Autodesk Inventor part; units mm, degrees
(part 2 of 16)
  spline S4 degree 3 poles (20.0299, 111.5354) (20.0063, 111.4026) (19.9809, 111.2702) (19.9533, 111.1381) (19.9384, 111.0668) (19.9228, 110.9955) (19.9066, 110.9244) (19.8913, 110.8571) (19.8754, 110.79) (19.8589, 110.723) (19.8433, 110.6597) (19.8272, 110.5966) (19.8105, 110.5336) (19.7948, 110.4744) (19.7786, 110.4154) (19.7618, 110.3565) (19.7461, 110.3013) (19.7299, 110.2462) (19.7133, 110.1914) (19.6977, 110.1402) (19.6817, 110.0892) (19.6653, 110.0383) (19.65, 109.9911) (19.6344, 109.944) (19.6183, 109.8971) (19.6035, 109.8539) (19.5883, 109.8108) (19.5727, 109.7678) (19.5584, 109.7285) (19.5438, 109.6893) (19.5288, 109.6503) (19.5152, 109.6149) (19.5014, 109.5795) (19.4872, 109.5444) (19.4744, 109.5128) (19.4614, 109.4813) (19.4481, 109.45) (19.4305, 109.4086) (19.4123, 109.3675) (19.3937, 109.3265) (19.3896, 109.3173) (19.3854, 109.3081) (19.3813, 109.2989) (19.3774, 109.2899) (19.3735, 109.2809) (19.3697, 109.2718) (19.366, 109.2629) (19.3623, 109.254) (19.3587, 109.2451) (19.3552, 109.2363) (19.3518, 109.2275) (19.3485, 109.2187) (19.3452, 109.21) (19.342, 109.2013) (19.3389, 109.1926) (19.3359, 109.184) (19.3329, 109.1753) (19.3301, 109.1667) (19.3273, 109.1581) (19.3245, 109.1496) (19.3219, 109.1409) (19.3193, 109.1324) (19.3168, 109.1238) (19.3144, 109.1152) (19.3121, 109.1067) (19.3098, 109.0981) (19.3077, 109.0895) (19.3055, 109.0808) (19.3035, 109.0721) (19.3017, 109.0634) (19.2998, 109.0546) (19.298, 109.0458) (19.2964, 109.037) (19.2948, 109.028) (19.2933, 109.019) (19.292, 109.0099) (19.2907, 109.0006) (19.2895, 108.9912) (19.2886, 108.9819) (19.2876, 108.9721) (19.2868, 108.9623) (19.2863, 108.9526) (19.2857, 108.9422) (19.2854, 108.9319) (19.2854, 108.9216) (19.2854, 108.9105) (19.2857, 108.8994) (19.2864, 108.8884) (19.2871, 108.8764) (19.2882, 108.8644) (19.2898, 108.8524) (19.2915, 108.8393) (19.2937, 108.8262) (19.2965, 108.8132) (19.2996, 108.7987) (19.3034, 108.7844) (19.3079, 108.7703) (19.3129, 108.7544) (19.3188, 108.7388) (19.3256, 108.7236) (19.3332, 108.7064) (19.3419, 108.6898) (19.3516, 108.6738) (19.3625, 108.6561) (19.3746, 108.6391) (19.3879, 108.6231) (19.4023, 108.6057) (19.4181, 108.5894) (19.4352, 108.5747) (19.4515, 108.5607) (19.469, 108.5481) (19.4867, 108.5358) (19.5744, 108.4751) (19.6668, 108.4221) (19.7564, 108.3646) (19.8461, 108.3071) (19.9329, 108.2453) (20.0247, 108.191) (20.0432, 108.18) (20.062, 108.1693) (20.0815, 108.1603) (20.102, 108.151) (20.1234, 108.1434) (20.1452, 108.1376) (20.1653, 108.1322) (20.1858, 108.1282) (20.2065, 108.1258) (20.225, 108.1236) (20.2438, 108.1227) (20.2625, 108.1229) (20.2792, 108.1231) (20.2958, 108.1243) (20.3123, 108.1263) (20.327, 108.1281) (20.3416, 108.1307) (20.3561, 108.1339) (20.3691, 108.1368) (20.3819, 108.1402) (20.3946, 108.1442) (20.4061, 108.1477) (20.4174, 108.1517) (20.4286, 108.1561) (20.4389, 108.1601) (20.4491, 108.1644) (20.4592, 108.1691) (20.4686, 108.1734) (20.4779, 108.178) (20.487, 108.1828) (20.4957, 108.1874) (20.5042, 108.1921) (20.5127, 108.1971) (20.5208, 108.2019) (20.5288, 108.2068) (20.5367, 108.2119) (20.5444, 108.2169) (20.552, 108.222) (20.5595, 108.2272) (20.5669, 108.2324) (20.5741, 108.2376) (20.5813, 108.243) (20.5885, 108.2484) (20.5955, 108.2538) (20.6025, 108.2594) (20.6094, 108.2649) (20.6163, 108.2706) (20.6231, 108.2763) (20.6299, 108.282) (20.6366, 108.2879) (20.6433, 108.2938) (20.6501, 108.2998) (20.6567, 108.3058) (20.6633, 108.312) (20.67, 108.3182) (20.6766, 108.3245) (20.6831, 108.3308) (20.6898, 108.3373) (20.6963, 108.3438) (20.7029, 108.3504) (20.7095, 108.3571) (20.7161, 108.3639) (20.7226, 108.3707) (20.7292, 108.3777) (20.7358, 108.3847) (20.7423, 108.3918) (20.7489, 108.3991) (20.7555, 108.4064) (20.7621, 108.4137) (20.7687, 108.4213) (20.7753, 108.4289) (20.7819, 108.4365) (20.8114, 108.4704) (20.8412, 108.5042) (20.8715, 108.5375) (20.8944, 108.5627) (20.9176, 108.5876) (20.9409, 108.6124) (20.967, 108.6399) (20.9933, 108.6673) (21.0198, 108.6944) (21.049, 108.7243) (21.0785, 108.754) (21.1083, 108.7833) (21.1408, 108.8154) (21.1737, 108.8472) (21.2067, 108.8788) (21.2427, 108.913) (21.2789, 108.9468) (21.3154, 108.9804) (21.3548, 109.0166) (21.3945, 109.0524) (21.4345, 109.0879) (21.4774, 109.126) (21.5207, 109.1636) (21.5642, 109.2009) (21.6108, 109.2408) (21.6577, 109.2801) (21.7049, 109.3191) (21.7552, 109.3606) (21.8058, 109.4016) (21.8567, 109.4422) (21.9108, 109.4851) (21.9652, 109.5276) (22.0199, 109.5696) (22.0778, 109.614) (22.136, 109.6579) (22.1946, 109.7012) (22.3031, 109.7814) (22.4128, 109.8598) (22.5237, 109.9366) knots 0 0 0 0 0.057795 0.057795 0.057795 0.089038 0.089038 0.089038 0.118617 0.118617 0.118617 0.14653 0.14653 0.14653 0.172778 0.172778 0.172778 0.19736 0.19736 0.19736 0.220277 0.220277 0.220277 0.241529 0.241529 0.241529 0.261115 0.261115 0.261115 0.279036 0.279036 0.279036 0.295292 0.295292 0.295292 0.309882 0.309882 0.309882 0.329164 0.329164 0.329164 0.333477 0.333477 0.333477 0.337694 0.337694 0.337694 0.34182 0.34182 0.34182 0.345864 0.345864 0.345864 0.349834 0.349834 0.349834 0.353742 0.353742 0.353742 0.3576 0.3576 0.3576 0.361424 0.361424 0.361424 0.365232 0.365232 0.365232 0.369048 0.369048 0.369048 0.372899 0.372899 0.372899 0.376819 0.376819 0.376819 0.380853 0.380853 0.380853 0.385052 0.385052 0.385052 0.389482 0.389482 0.389482 0.394225 0.394225 0.394225 0.399381 0.399381 0.399381 0.405067 0.405067 0.405067 0.411413 0.411413 0.411413 0.418548 0.418548 0.418548 0.426565 0.426565 0.426565 0.435472 0.435472 0.435472 0.445133 0.445133 0.445133 0.45436 0.45436 0.45436 0.5 0.5 0.5 0.54564 0.54564 0.54564 0.554867 0.554867 0.554867 0.564528 0.564528 0.564528 0.573435 0.573435 0.573435 0.581452 0.581452 0.581452 0.588587 0.588587 0.588587 0.594933 0.594933 0.594933 0.600619 0.600619 0.600619 0.605775 0.605775 0.605775 0.610518 0.610518 0.610518 0.614948 0.614948 0.614948 0.619147 0.619147 0.619147 0.623181 0.623181 0.623181 0.627101 0.627101 0.627101 0.630952 0.630952 0.630952 0.634768 0.634768 0.634768 0.638576 0.638576 0.638576 0.6424 0.6424 0.6424 0.646258 0.646258 0.646258 0.650166 0.650166 0.650166 0.654136 0.654136 0.654136 0.65818 0.65818 0.65818 0.662306 0.662306 0.662306 0.666523 0.666523 0.666523 0.670836 0.670836 0.670836 0.690118 0.690118 0.690118 0.704708 0.704708 0.704708 0.720964 0.720964 0.720964 0.738885 0.738885 0.738885 0.758471 0.758471 0.758471 0.779723 0.779723 0.779723 0.80264 0.80264 0.80264 0.827222 0.827222 0.827222 0.85347 0.85347 0.85347 0.881383 0.881383 0.881383 0.910962 0.910962 0.910962 0.942205 0.942205 0.942205 1 1 1 1
  arc A206 (20.0299, 111.5354) -> (19.0221, 112.1094) centre (0.0435, 77.6158) ccw
  spline S5 degree 3 poles (16.3748, 113.4387) (16.3653, 113.3042) (16.3538, 113.1698) (16.3402, 113.0356) (16.3328, 112.9631) (16.3248, 112.8906) (16.3161, 112.8182) (16.3079, 112.7497) (16.2991, 112.6812) (16.2897, 112.6129) (16.2808, 112.5483) (16.2714, 112.4839) (16.2614, 112.4195) (16.2519, 112.359) (16.242, 112.2986) (16.2315, 112.2382) (16.2216, 112.1817) (16.2113, 112.1253) (16.2004, 112.069) (16.1903, 112.0164) (16.1798, 111.964) (16.1687, 111.9117) (16.1585, 111.8632) (16.1478, 111.8147) (16.1367, 111.7664) (16.1265, 111.7219) (16.1159, 111.6774) (16.1049, 111.633) (16.0948, 111.5925) (16.0844, 111.552) (16.0736, 111.5116) (16.0638, 111.4749) (16.0536, 111.4384) (16.0432, 111.4019) (16.0338, 111.3692) (16.0242, 111.3365) (16.0142, 111.3039) (16.001, 111.2609) (15.9872, 111.2181) (15.9731, 111.1754) (15.9699, 111.1658) (15.9667, 111.1563) (15.9636, 111.1467) (15.9606, 111.1373) (15.9577, 111.1279) (15.9549, 111.1185) (15.9521, 111.1093) (15.9494, 111.1001) (15.9468, 111.0908) (15.9442, 111.0817) (15.9417, 111.0726) (15.9393, 111.0635) (15.937, 111.0545) (15.9347, 111.0455) (15.9326, 111.0365) (15.9304, 111.0276) (15.9284, 111.0188) (15.9265, 111.0098) (15.9246, 111.0011) (15.9227, 110.9922) (15.921, 110.9834) (15.9193, 110.9746) (15.9178, 110.9658) (15.9163, 110.957) (15.9148, 110.9483) (15.9135, 110.9395) (15.9123, 110.9307) (15.911, 110.9219) (15.9099, 110.913) (15.909, 110.9042) (15.908, 110.8952) (15.9072, 110.8863) (15.9065, 110.8773) (15.9058, 110.8682) (15.9053, 110.8591) (15.905, 110.8499) (15.9046, 110.8405) (15.9045, 110.8311) (15.9045, 110.8217) (15.9045, 110.8119) (15.9048, 110.8021) (15.9053, 110.7923) (15.9058, 110.782) (15.9066, 110.7717) (15.9077, 110.7614) (15.9088, 110.7504) (15.9103, 110.7394) (15.9121, 110.7285) (15.9141, 110.7166) (15.9164, 110.7048) (15.9192, 110.6931) (15.9223, 110.6802) (15.9259, 110.6674) (15.93, 110.6548) (15.9346, 110.6407) (15.9399, 110.6268) (15.9458, 110.6133) (15.9525, 110.598) (15.96, 110.5831) (15.9683, 110.5687) (15.9777, 110.5524) (15.988, 110.5368) (15.9994, 110.5219) (16.012, 110.5054) (16.0259, 110.4898) (16.0408, 110.4753) (16.0569, 110.4595) (16.0743, 110.445) (16.0928, 110.4321) (16.1105, 110.4199) (16.1293, 110.4092) (16.1482, 110.3988) (16.2417, 110.3476) (16.3392, 110.3045) (16.4343, 110.2567) (16.5295, 110.2089) (16.6223, 110.1565) (16.7192, 110.1121) (16.7388, 110.1031) (16.7586, 110.0944) (16.779, 110.0876) (16.8003, 110.0804) (16.8224, 110.0751) (16.8447, 110.0716) (16.8653, 110.0683) (16.886, 110.0665) (16.9068, 110.0663) (16.9255, 110.066) (16.9443, 110.067) (16.9629, 110.0692) (16.9794, 110.0712) (16.9959, 110.0741) (17.0121, 110.0778) (17.0265, 110.0812) (17.0408, 110.0853) (17.0548, 110.09) (17.0674, 110.0942) (17.0798, 110.099) (17.092, 110.1042) (17.103, 110.1089) (17.1139, 110.1141) (17.1246, 110.1196) (17.1345, 110.1247) (17.1442, 110.1301) (17.1537, 110.1357) (17.1626, 110.141) (17.1713, 110.1465) (17.1799, 110.1523) (17.188, 110.1577) (17.196, 110.1634) (17.2039, 110.1692) (17.2115, 110.1748) (17.219, 110.1805) (17.2263, 110.1864) (17.2334, 110.1922) (17.2404, 110.198) (17.2473, 110.204) (17.2541, 110.2099) (17.2608, 110.2159) (17.2674, 110.222) (17.2739, 110.2281) (17.2804, 110.2343) (17.2867, 110.2405) (17.2931, 110.2467) (17.2993, 110.2531) (17.3054, 110.2595) (17.3116, 110.2659) (17.3177, 110.2724) (17.3237, 110.279) (17.3298, 110.2857) (17.3358, 110.2924) (17.3417, 110.2992) (17.3477, 110.306) (17.3536, 110.313) (17.3595, 110.32) (17.3654, 110.3271) (17.3713, 110.3343) (17.377, 110.3415) (17.3829, 110.3489) (17.3888, 110.3563) (17.3945, 110.3638) (17.4004, 110.3714) (17.4062, 110.3791) (17.4119, 110.3868) (17.4178, 110.3948) (17.4236, 110.4027) (17.4293, 110.4107) (17.4351, 110.4189) (17.4409, 110.4272) (17.4467, 110.4354) (17.4725, 110.4723) (17.4986, 110.5089) (17.5252, 110.5452) (17.5453, 110.5726) (17.5658, 110.5999) (17.5864, 110.6269) (17.6094, 110.6571) (17.6327, 110.687) (17.6563, 110.7168) (17.6822, 110.7496) (17.7085, 110.7821) (17.735, 110.8145) (17.764, 110.8498) (17.7933, 110.8849) (17.8229, 110.9197) (17.8551, 110.9574) (17.8876, 110.9949) (17.9204, 111.0321) (17.9557, 111.0722) (17.9915, 111.112) (18.0276, 111.1515) (18.0663, 111.1938) (18.1054, 111.2358) (18.1448, 111.2774) (18.1869, 111.3219) (18.2295, 111.366) (18.2724, 111.4097) (18.318, 111.4562) (18.364, 111.5022) (18.4105, 111.5479) (18.4597, 111.5963) (18.5094, 111.6442) (18.5594, 111.6918) (18.6123, 111.7419) (18.6657, 111.7916) (18.7195, 111.8409) (18.8189, 111.9319) (18.9198, 112.0214) (19.0221, 112.1094) knots 0 0 0 0 0.057795 0.057795 0.057795 0.089038 0.089038 0.089038 0.118617 0.118617 0.118617 0.14653 0.14653 0.14653 0.172778 0.172778 0.172778 0.19736 0.19736 0.19736 0.220277 0.220277 0.220277 0.241529 0.241529 0.241529 0.261115 0.261115 0.261115 0.279036 0.279036 0.279036 0.295292 0.295292 0.295292 0.309882 0.309882 0.309882 0.329164 0.329164 0.329164 0.333477 0.333477 0.333477 0.337694 0.337694 0.337694 0.34182 0.34182 0.34182 0.345864 0.345864 0.345864 0.349834 0.349834 0.349834 0.353742 0.353742 0.353742 0.3576 0.3576 0.3576 0.361424 0.361424 0.361424 0.365232 0.365232 0.365232 0.369048 0.369048 0.369048 0.372899 0.372899 0.372899 0.376819 0.376819 0.376819 0.380853 0.380853 0.380853 0.385052 0.385052 0.385052 0.389482 0.389482 0.389482 0.394225 0.394225 0.394225 0.399381 0.399381 0.399381 0.405067 0.405067 0.405067 0.411413 0.411413 0.411413 0.418548 0.418548 0.418548 0.426565 0.426565 0.426565 0.435472 0.435472 0.435472 0.445133 0.445133 0.445133 0.45436 0.45436 0.45436 0.5 0.5 0.5 0.54564 0.54564 0.54564 0.554867 0.554867 0.554867 0.564528 0.564528 0.564528 0.573435 0.573435 0.573435 0.581452 0.581452 0.581452 0.588587 0.588587 0.588587 0.594933 0.594933 0.594933 0.600619 0.600619 0.600619 0.605775 0.605775 0.605775 0.610518 0.610518 0.610518 0.614948 0.614948 0.614948 0.619147 0.619147 0.619147 0.623181 0.623181 0.623181 0.627101 0.627101 0.627101 0.630952 0.630952 0.630952 0.634768 0.634768 0.634768 0.638576 0.638576 0.638576 0.6424 0.6424 0.6424 0.646258 0.646258 0.646258 0.650166 0.650166 0.650166 0.654136 0.654136 0.654136 0.65818 0.65818 0.65818 0.662306 0.662306 0.662306 0.666523 0.666523 0.666523 0.670836 0.670836 0.670836 0.690118 0.690118 0.690118 0.704708 0.704708 0.704708 0.720964 0.720964 0.720964 0.738885 0.738885 0.738885 0.758471 0.758471 0.758471 0.779723 0.779723 0.779723 0.80264 0.80264 0.80264 0.827222 0.827222 0.827222 0.85347 0.85347 0.85347 0.881383 0.881383 0.881383 0.910962 0.910962 0.910962 0.942205 0.942205 0.942205 1 1 1 1
  arc A207 (16.3748, 113.4387) -> (15.3125, 113.9042) centre (0.0435, 77.6158) ccw
  spline S6 degree 3 poles (12.5408, 114.9496) (12.5454, 114.8148) (12.548, 114.6799) (12.5485, 114.5451) (12.5488, 114.4722) (12.5484, 114.3993) (12.5473, 114.3264) (12.5463, 114.2573) (12.5447, 114.1883) (12.5425, 114.1193) (12.5404, 114.0542) (12.5378, 113.9892) (12.5345, 113.9241) (12.5315, 113.8629) (12.5279, 113.8018) (12.5237, 113.7407) (12.5199, 113.6834) (12.5155, 113.6262) (12.5106, 113.5691) (12.506, 113.5158) (12.501, 113.4626) (12.4955, 113.4094) (12.4904, 113.36) (12.4849, 113.3108) (12.4789, 113.2615) (12.4733, 113.2162) (12.4674, 113.1708) (12.4611, 113.1256) (12.4553, 113.0841) (12.4492, 113.0428) (12.4427, 113.0015) (12.4368, 112.964) (12.4305, 112.9266) (12.4239, 112.8892) (12.418, 112.8557) (12.4119, 112.8222) (12.4053, 112.7888) (12.3967, 112.7446) (12.3875, 112.7006) (12.3779, 112.6566) (12.3757, 112.6468) (12.3735, 112.637) (12.3715, 112.6271) (12.3695, 112.6175) (12.3675, 112.6078) (12.3657, 112.5982) (12.3639, 112.5887) (12.3622, 112.5792) (12.3606, 112.5698) (12.359, 112.5605) (12.3574, 112.5511) (12.356, 112.5418) (12.3546, 112.5327) (12.3533, 112.5235) (12.3521, 112.5143) (12.3509, 112.5053) (12.3498, 112.4962) (12.3488, 112.4871) (12.3478, 112.4782) (12.347, 112.4692) (12.3462, 112.4603) (12.3454, 112.4514) (12.3448, 112.4425) (12.3442, 112.4336) (12.3437, 112.4247) (12.3433, 112.4158) (12.343, 112.4069) (12.3427, 112.398) (12.3425, 112.3891) (12.3425, 112.3802) (12.3425, 112.3712) (12.3426, 112.3622) (12.3428, 112.3533) (12.3431, 112.3441) (12.3436, 112.335) (12.3442, 112.3259) (12.3448, 112.3165) (12.3456, 112.3071) (12.3467, 112.2977) (12.3477, 112.288) (12.349, 112.2783) (12.3505, 112.2686) (12.3521, 112.2584) (12.354, 112.2482) (12.3561, 112.2381) (12.3584, 112.2272) (12.361, 112.2165) (12.3639, 112.2058) (12.3671, 112.1942) (12.3707, 112.1827) (12.3747, 112.1714) (12.3791, 112.1589) (12.3841, 112.1465) (12.3895, 112.1344) (12.3955, 112.1209) (12.4022, 112.1076) (12.4095, 112.0947) (12.4177, 112.0803) (12.4268, 112.0662) (12.4365, 112.0527) (12.4475, 112.0376) (12.4595, 112.0231) (12.4724, 112.0095) (12.4866, 111.9944) (12.502, 111.9803) (12.5184, 111.9674) (12.5361, 111.9534) (12.5549, 111.9408) (12.5747, 111.93) (12.5936, 111.9196) (12.6133, 111.911) (12.6332, 111.9026) (12.7316, 111.8615) (12.833, 111.8288) (12.9326, 111.7912) (13.0323, 111.7536) (13.13, 111.7112) (13.2311, 111.6772) (13.2515, 111.6703) (13.2721, 111.6637) (13.2931, 111.659) (13.3151, 111.6541) (13.3376, 111.6512) (13.3601, 111.65) (13.3809, 111.6489) (13.4017, 111.6493) (13.4225, 111.6512) (13.4411, 111.6529) (13.4596, 111.6559) (13.4779, 111.66) (13.4941, 111.6637) (13.5102, 111.6683) (13.5259, 111.6737) (13.5399, 111.6786) (13.5537, 111.6841) (13.5671, 111.6902) (13.5792, 111.6958) (13.5911, 111.7018) (13.6026, 111.7083) (13.6131, 111.7141) (13.6234, 111.7204) (13.6335, 111.727) (13.6427, 111.7331) (13.6518, 111.7394) (13.6607, 111.7461) (13.669, 111.7523) (13.6771, 111.7587) (13.685, 111.7653) (13.6926, 111.7715) (13.6999, 111.778) (13.7072, 111.7846) (13.7141, 111.791) (13.7209, 111.7975) (13.7276, 111.8041) (13.7341, 111.8105) (13.7405, 111.8171) (13.7467, 111.8238) (13.7528, 111.8304) (13.7589, 111.837) (13.7648, 111.8438) (13.7706, 111.8505) (13.7764, 111.8573) (13.782, 111.8642) (13.7877, 111.871) (13.7932, 111.878) (13.7987, 111.885) (13.8042, 111.8921) (13.8095, 111.8992) (13.8148, 111.9064) (13.8202, 111.9136) (13.8254, 111.9209) (13.8306, 111.9283) (13.8359, 111.9357) (13.841, 111.9433) (13.8461, 111.9508) (13.8512, 111.9585) (13.8563, 111.9663) (13.8613, 111.9741) (13.8664, 111.982) (13.8714, 111.99) (13.8764, 111.9981) (13.8814, 112.0063) (13.8864, 112.0145) (13.8913, 112.0228) (13.8963, 112.0313) (13.9012, 112.0398) (13.9061, 112.0484) (13.911, 112.0571) (13.9159, 112.0659) (13.9208, 112.0747) (13.9426, 112.1141) (13.9647, 112.1533) (13.9874, 112.1921) (14.0045, 112.2215) (14.022, 112.2508) (14.0397, 112.2798) (14.0595, 112.3122) (14.0795, 112.3445) (14.0998, 112.3765) (14.1222, 112.4118) (14.1449, 112.4469) (14.1679, 112.4819) (14.193, 112.52) (14.2185, 112.558) (14.2443, 112.5957) (14.2723, 112.6366) (14.3007, 112.6773) (14.3295, 112.7177) (14.3605, 112.7613) (14.3919, 112.8046) (14.4236, 112.8476) (14.4577, 112.8938) (14.4922, 112.9396) (14.527, 112.9851) (14.5643, 113.0338) (14.602, 113.082) (14.6401, 113.13) (14.6806, 113.181) (14.7216, 113.2316) (14.763, 113.2819) (14.8069, 113.3352) (14.8513, 113.388) (14.8961, 113.4405) (14.9435, 113.496) (14.9913, 113.551) (15.0396, 113.6055) (15.1291, 113.7065) (15.2201, 113.8061) (15.3125, 113.9042) knots 0 0 0 0 0.057795 0.057795 0.057795 0.089038 0.089038 0.089038 0.118617 0.118617 0.118617 0.14653 0.14653 0.14653 0.172778 0.172778 0.172778 0.19736 0.19736 0.19736 0.220277 0.220277 0.220277 0.241529 0.241529 0.241529 0.261115 0.261115 0.261115 0.279036 0.279036 0.279036 0.295292 0.295292 0.295292 0.309882 0.309882 0.309882 0.329164 0.329164 0.329164 0.333477 0.333477 0.333477 0.337694 0.337694 0.337694 0.34182 0.34182 0.34182 0.345864 0.345864 0.345864 0.349834 0.349834 0.349834 0.353742 0.353742 0.353742 0.3576 0.3576 0.3576 0.361424 0.361424 0.361424 0.365232 0.365232 0.365232 0.369048 0.369048 0.369048 0.372899 0.372899 0.372899 0.376819 0.376819 0.376819 0.380853 0.380853 0.380853 0.385052 0.385052 0.385052 0.389482 0.389482 0.389482 0.394225 0.394225 0.394225 0.399381 0.399381 0.399381 0.405067 0.405067 0.405067 0.411413 0.411413 0.411413 0.418548 0.418548 0.418548 0.426565 0.426565 0.426565 0.435472 0.435472 0.435472 0.445133 0.445133 0.445133 0.45436 0.45436 0.45436 0.5 0.5 0.5 0.54564 0.54564 0.54564 0.554867 0.554867 0.554867 0.564528 0.564528 0.564528 0.573435 0.573435 0.573435 0.581452 0.581452 0.581452 0.588587 0.588587 0.588587 0.594933 0.594933 0.594933 0.600619 0.600619 0.600619 0.605775 0.605775 0.605775 0.610518 0.610518 0.610518 0.614948 0.614948 0.614948 0.619147 0.619147 0.619147 0.623181 0.623181 0.623181 0.627101 0.627101 0.627101 0.630952 0.630952 0.630952 0.634768 0.634768 0.634768 0.638576 0.638576 0.638576 0.6424 0.6424 0.6424 0.646258 0.646258 0.646258 0.650166 0.650166 0.650166 0.654136 0.654136 0.654136 0.65818 0.65818 0.65818 0.662306 0.662306 0.662306 0.666523 0.666523 0.666523 0.670836 0.670836 0.670836 0.690118 0.690118 0.690118 0.704708 0.704708 0.704708 0.720964 0.720964 0.720964 0.738885 0.738885 0.738885 0.758471 0.758471 0.758471 0.779723 0.779723 0.779723 0.80264 0.80264 0.80264 0.827222 0.827222 0.827222 0.85347 0.85347 0.85347 0.881383 0.881383 0.881383 0.910962 0.910962 0.910962 0.942205 0.942205 0.942205 1 1 1 1
  arc A208 (12.5408, 114.9496) -> (11.4357, 115.3015) centre (0.0435, 77.6158) ccw
  spline S7 degree 3 poles (8.5699, 116.0514) (8.5886, 115.9178) (8.6053, 115.784) (8.6198, 115.6499) (8.6277, 115.5774) (8.635, 115.5049) (8.6415, 115.4323) (8.6478, 115.3635) (8.6534, 115.2947) (8.6584, 115.2259) (8.6631, 115.1609) (8.6673, 115.0959) (8.6709, 115.0309) (8.6742, 114.9697) (8.677, 114.9085) (8.6793, 114.8473) (8.6814, 114.79) (8.6831, 114.7326) (8.6842, 114.6753) (8.6852, 114.6218) (8.6858, 114.5684) (8.6858, 114.5149) (8.6859, 114.4653) (8.6856, 114.4157) (8.6847, 114.3661) (8.684, 114.3204) (8.6829, 114.2747) (8.6813, 114.229) (8.6799, 114.1872) (8.6781, 114.1455) (8.6759, 114.1037) (8.674, 114.0658) (8.6717, 114.0279) (8.669, 113.9901) (8.6667, 113.9561) (8.664, 113.9222) (8.661, 113.8883) (8.6571, 113.8435) (8.6525, 113.7987) (8.6475, 113.754) (8.6464, 113.744) (8.6453, 113.734) (8.6443, 113.724) (8.6433, 113.7142) (8.6424, 113.7044) (8.6416, 113.6946) (8.6408, 113.685) (8.64, 113.6754) (8.6394, 113.6658) (8.6388, 113.6563) (8.6383, 113.6469) (8.6378, 113.6375) (8.6374, 113.6282) (8.637, 113.619) (8.6368, 113.6097) (8.6366, 113.6006) (8.6364, 113.5915) (8.6364, 113.5824) (8.6363, 113.5734) (8.6364, 113.5644) (8.6366, 113.5554) (8.6367, 113.5464) (8.637, 113.5375) (8.6374, 113.5286) (8.6378, 113.5197) (8.6383, 113.5108) (8.6389, 113.502) (8.6396, 113.4931) (8.6403, 113.4842) (8.6412, 113.4754) (8.6421, 113.4664) (8.6432, 113.4575) (8.6444, 113.4486) (8.6456, 113.4395) (8.647, 113.4305) (8.6486, 113.4215) (8.6502, 113.4122) (8.652, 113.403) (8.654, 113.3938) (8.6561, 113.3842) (8.6584, 113.3747) (8.6609, 113.3652) (8.6635, 113.3552) (8.6665, 113.3453) (8.6696, 113.3354) (8.6731, 113.3249) (8.6768, 113.3145) (8.6808, 113.3042) (8.6852, 113.293) (8.69, 113.2819) (8.6951, 113.271) (8.7008, 113.259) (8.707, 113.2473) (8.7137, 113.2358) (8.7211, 113.223) (8.7291, 113.2105) (8.7378, 113.1985) (8.7474, 113.1849) (8.7579, 113.1719) (8.769, 113.1595) (8.7815, 113.1456) (8.7949, 113.1325) (8.8091, 113.1203) (8.8249, 113.1067) (8.8417, 113.0944) (8.8593, 113.0832) (8.8784, 113.0712) (8.8984, 113.0605) (8.9192, 113.0519) (8.9391, 113.0436) (8.9596, 113.037) (8.9803, 113.0308) (9.0824, 113.0001) (9.1867, 112.9782) (9.2897, 112.9513) (9.3927, 112.9243) (9.4944, 112.8923) (9.5985, 112.869) (9.6195, 112.8643) (9.6406, 112.86) (9.662, 112.8575) (9.6844, 112.8549) (9.7071, 112.8543) (9.7296, 112.8555) (9.7504, 112.8566) (9.7711, 112.8592) (9.7915, 112.8632) (9.8098, 112.8669) (9.828, 112.8718) (9.8457, 112.8778) (9.8615, 112.8831) (9.8769, 112.8894) (9.892, 112.8964) (9.9054, 112.9027) (9.9186, 112.9097) (9.9313, 112.9172) (9.9427, 112.9239) (9.9539, 112.9312) (9.9647, 112.9388) (9.9745, 112.9458) (9.9841, 112.9531) (9.9934, 112.9607) (10.002, 112.9677) (10.0104, 112.975) (10.0185, 112.9825) (10.0261, 112.9895) (10.0335, 112.9967) (10.0407, 113.0041) (10.0475, 113.0112) (10.0542, 113.0183) (10.0607, 113.0257) (10.0669, 113.0327) (10.073, 113.0399) (10.079, 113.0472) (10.0848, 113.0543) (10.0904, 113.0615) (10.0959, 113.0688) (10.1013, 113.076) (10.1066, 113.0832) (10.1118, 113.0906) (10.1169, 113.0978) (10.1219, 113.1052) (10.1269, 113.1126) (10.1317, 113.1201) (10.1365, 113.1275) (10.1412, 113.1351) (10.1459, 113.1427) (10.1505, 113.1503) (10.1551, 113.158) (10.1596, 113.1658) (10.1641, 113.1736) (10.1685, 113.1815) (10.1729, 113.1894) (10.1772, 113.1975) (10.1815, 113.2055) (10.1858, 113.2137) (10.19, 113.222) (10.1942, 113.2302) (10.1984, 113.2387) (10.2026, 113.2471) (10.2067, 113.2557) (10.2108, 113.2643) (10.2149, 113.2731) (10.2189, 113.2818) (10.223, 113.2908) (10.227, 113.2998) (10.2309, 113.3088) (10.2349, 113.318) (10.2389, 113.3273) (10.2428, 113.3365) (10.2604, 113.378) (10.2783, 113.4192) (10.2968, 113.4603) (10.3108, 113.4913) (10.3251, 113.5222) (10.3397, 113.5529) (10.3559, 113.5872) (10.3725, 113.6214) (10.3893, 113.6554) (10.4079, 113.6928) (10.4268, 113.7301) (10.446, 113.7673) (10.467, 113.8079) (10.4884, 113.8482) (10.5101, 113.8885) (10.5337, 113.9321) (10.5577, 113.9755) (10.5821, 114.0187) (10.6083, 114.0653) (10.635, 114.1116) (10.6621, 114.1577) (10.6912, 114.2072) (10.7207, 114.2564) (10.7506, 114.3053) (10.7826, 114.3576) (10.815, 114.4095) (10.8479, 114.4612) (10.8828, 114.5162) (10.9183, 114.5708) (10.9542, 114.6251) (10.9923, 114.6827) (11.0309, 114.7399) (11.07, 114.7968) (11.1113, 114.8569) (11.1532, 114.9166) (11.1955, 114.9759) (11.2739, 115.0857) (11.354, 115.1942) (11.4357, 115.3015) knots 0 0 0 0 0.057795 0.057795 0.057795 0.089038 0.089038 0.089038 0.118617 0.118617 0.118617 0.14653 0.14653 0.14653 0.172778 0.172778 0.172778 0.19736 0.19736 0.19736 0.220277 0.220277 0.220277 0.241529 0.241529 0.241529 0.261115 0.261115 0.261115 0.279036 0.279036 0.279036 0.295292 0.295292 0.295292 0.309882 0.309882 0.309882 0.329164 0.329164 0.329164 0.333477 0.333477 0.333477 0.337694 0.337694 0.337694 0.34182 0.34182 0.34182 0.345864 0.345864 0.345864 0.349834 0.349834 0.349834 0.353742 0.353742 0.353742 0.3576 0.3576 0.3576 0.361424 0.361424 0.361424 0.365232 0.365232 0.365232 0.369048 0.369048 0.369048 0.372899 0.372899 0.372899 0.376819 0.376819 0.376819 0.380853 0.380853 0.380853 0.385052 0.385052 0.385052 0.389482 0.389482 0.389482 0.394225 0.394225 0.394225 0.399381 0.399381 0.399381 0.405067 0.405067 0.405067 0.411413 0.411413 0.411413 0.418548 0.418548 0.418548 0.426565 0.426565 0.426565 0.435472 0.435472 0.435472 0.445133 0.445133 0.445133 0.45436 0.45436 0.45436 0.5 0.5 0.5 0.54564 0.54564 0.54564 0.554867 0.554867 0.554867 0.564528 0.564528 0.564528 0.573435 0.573435 0.573435 0.581452 0.581452 0.581452 0.588587 0.588587 0.588587 0.594933 0.594933 0.594933 0.600619 0.600619 0.600619 0.605775 0.605775 0.605775 0.610518 0.610518 0.610518 0.614948 0.614948 0.614948 0.619147 0.619147 0.619147 0.623181 0.623181 0.623181 0.627101 0.627101 0.627101 0.630952 0.630952 0.630952 0.634768 0.634768 0.634768 0.638576 0.638576 0.638576 0.6424 0.6424 0.6424 0.646258 0.646258 0.646258 0.650166 0.650166 0.650166 0.654136 0.654136 0.654136 0.65818 0.65818 0.65818 0.662306 0.662306 0.662306 0.666523 0.666523 0.666523 0.670836 0.670836 0.670836 0.690118 0.690118 0.690118 0.704708 0.704708 0.704708 0.720964 0.720964 0.720964 0.738885 0.738885 0.738885 0.758471 0.758471 0.758471 0.779723 0.779723 0.779723 0.80264 0.80264 0.80264 0.827222 0.827222 0.827222 0.85347 0.85347 0.85347 0.881383 0.881383 0.881383 0.910962 0.910962 0.910962 0.942205 0.942205 0.942205 1 1 1 1
  arc A209 (8.5699, 116.0514) -> (7.4341, 116.2859) centre (0.0435, 77.6158) ccw
  spline S8 degree 3 poles (4.5056, 116.7321) (4.5381, 116.6012) (4.5687, 116.4698) (4.5972, 116.338) (4.6126, 116.2668) (4.6274, 116.1954) (4.6415, 116.1238) (4.6549, 116.0561) (4.6677, 115.9883) (4.6799, 115.9203) (4.6914, 115.8562) (4.7023, 115.792) (4.7126, 115.7277) (4.7224, 115.6672) (4.7316, 115.6067) (4.7402, 115.546) (4.7483, 115.4893) (4.756, 115.4324) (4.763, 115.3755) (4.7697, 115.3224) (4.7758, 115.2693) (4.7815, 115.2161) (4.7867, 115.1668) (4.7916, 115.1174) (4.796, 115.068) (4.8, 115.0225) (4.8036, 114.9769) (4.8069, 114.9314) (4.8098, 114.8896) (4.8124, 114.8479) (4.8146, 114.8061) (4.8166, 114.7683) (4.8183, 114.7304) (4.8196, 114.6925) (4.8208, 114.6584) (4.8218, 114.6244) (4.8223, 114.5904) (4.8231, 114.5454) (4.8232, 114.5004) (4.8229, 114.4554) (4.8229, 114.4453) (4.8228, 114.4352) (4.8228, 114.4252) (4.8228, 114.4153) (4.823, 114.4055) (4.8232, 114.3957) (4.8234, 114.386) (4.8237, 114.3764) (4.8241, 114.3668) (4.8244, 114.3574) (4.8249, 114.3479) (4.8254, 114.3385) (4.826, 114.3293) (4.8266, 114.32) (4.8273, 114.3108) (4.828, 114.3017) (4.8288, 114.2926) (4.8298, 114.2835) (4.8307, 114.2746) (4.8317, 114.2656) (4.8328, 114.2567) (4.8339, 114.2478) (4.8351, 114.239) (4.8364, 114.2302) (4.8377, 114.2214) (4.8391, 114.2126) (4.8407, 114.2039) (4.8423, 114.1951) (4.844, 114.1864) (4.8458, 114.1776) (4.8476, 114.1688) (4.8496, 114.1601) (4.8517, 114.1513) (4.8539, 114.1425) (4.8562, 114.1336) (4.8587, 114.1248) (4.8613, 114.1158) (4.8641, 114.1068) (4.867, 114.0978) (4.8701, 114.0885) (4.8734, 114.0793) (4.8769, 114.0701) (4.8805, 114.0605) (4.8845, 114.0509) (4.8887, 114.0414) (4.8932, 114.0313) (4.8979, 114.0213) (4.903, 114.0115) (4.9086, 114.0008) (4.9145, 113.9903) (4.9208, 113.9801) (4.9277, 113.9687) (4.935, 113.9577) (4.9429, 113.947) (4.9516, 113.935) (4.9609, 113.9234) (4.9707, 113.9123) (4.9818, 113.8999) (4.9935, 113.888) (5.0059, 113.8769) (5.0198, 113.8643) (5.0345, 113.8527) (5.0499, 113.842) (5.067, 113.8302) (5.085, 113.8197) (5.1036, 113.8104) (5.1239, 113.8004) (5.1449, 113.792) (5.1665, 113.7855) (5.1871, 113.7793) (5.2083, 113.7749) (5.2294, 113.7709) (5.3342, 113.7511) (5.4402, 113.7402) (5.5455, 113.7242) (5.6508, 113.7082) (5.7552, 113.687) (5.8612, 113.6747) (5.8826, 113.6722) (5.904, 113.6701) (5.9256, 113.6698) (5.9481, 113.6696) (5.9707, 113.6714) (5.993, 113.6749) (6.0136, 113.6782) (6.0339, 113.6829) (6.0537, 113.6891) (6.0716, 113.6947) (6.0891, 113.7014) (6.1061, 113.7092) (6.1212, 113.7162) (6.136, 113.724) (6.1502, 113.7326) (6.1629, 113.7403) (6.1752, 113.7485) (6.1871, 113.7574) (6.1978, 113.7653) (6.2081, 113.7736) (6.2181, 113.7824) (6.2272, 113.7903) (6.2359, 113.7986) (6.2444, 113.8071) (6.2522, 113.815) (6.2597, 113.8231) (6.267, 113.8314) (6.2738, 113.8392) (6.2804, 113.8471) (6.2868, 113.8553) (6.2929, 113.863) (6.2988, 113.8708) (6.3045, 113.8788) (6.31, 113.8864) (6.3153, 113.8942) (6.3204, 113.9021) (6.3254, 113.9097) (6.3303, 113.9175) (6.335, 113.9253) (6.3396, 113.933) (6.3441, 113.9408) (6.3485, 113.9487) (6.3529, 113.9564) (6.3571, 113.9643) (6.3612, 113.9722) (6.3653, 113.9801) (6.3693, 113.988) (6.3731, 113.996) (6.377, 114.004) (6.3808, 114.0121) (6.3845, 114.0203) (6.3882, 114.0284) (6.3918, 114.0367) (6.3954, 114.045) (6.3989, 114.0534) (6.4024, 114.0618) (6.4058, 114.0703) (6.4092, 114.0789) (6.4126, 114.0875) (6.4159, 114.0962) (6.4192, 114.105) (6.4224, 114.1139) (6.4256, 114.1228) (6.4288, 114.1318) (6.432, 114.1409) (6.435, 114.1501) (6.4382, 114.1594) (6.4412, 114.1687) (6.4442, 114.1781) (6.4472, 114.1877) (6.4501, 114.1974) (6.4531, 114.207) (6.4662, 114.25) (6.4797, 114.2929) (6.4938, 114.3357) (6.5045, 114.368) (6.5155, 114.4002) (6.5268, 114.4323) (6.5394, 114.4681) (6.5523, 114.5038) (6.5655, 114.5394) (6.58, 114.5786) (6.5949, 114.6176) (6.6102, 114.6566) (6.6268, 114.6991) (6.6439, 114.7416) (6.6613, 114.7838) (6.6802, 114.8297) (6.6995, 114.8753) (6.7192, 114.9208) (6.7404, 114.9699) (6.7621, 115.0188) (6.7843, 115.0675) (6.808, 115.1197) (6.8322, 115.1717) (6.8568, 115.2235) (6.8832, 115.2788) (6.91, 115.3339) (6.9373, 115.3887) (6.9663, 115.447) (6.9959, 115.5051) (7.0259, 115.5629) (7.0578, 115.6241) (7.0902, 115.685) (7.1231, 115.7457) (7.1579, 115.8098) (7.1933, 115.8735) (7.2292, 115.937) (7.2957, 116.0543) (7.364, 116.1706) (7.4341, 116.2859) knots 0 0 0 0 0.057795 0.057795 0.057795 0.089038 0.089038 0.089038 0.118617 0.118617 0.118617 0.14653 0.14653 0.14653 0.172778 0.172778 0.172778 0.19736 0.19736 0.19736 0.220277 0.220277 0.220277 0.241529 0.241529 0.241529 0.261115 0.261115 0.261115 0.279036 0.279036 0.279036 0.295292 0.295292 0.295292 0.309882 0.309882 0.309882 0.329164 0.329164 0.329164 0.333477 0.333477 0.333477 0.337694 0.337694 0.337694 0.34182 0.34182 0.34182 0.345864 0.345864 0.345864 0.349834 0.349834 0.349834 0.353742 0.353742 0.353742 0.3576 0.3576 0.3576 0.361424 0.361424 0.361424 0.365232 0.365232 0.365232 0.369048 0.369048 0.369048 0.372899 0.372899 0.372899 0.376819 0.376819 0.376819 0.380853 0.380853 0.380853 0.385052 0.385052 0.385052 0.389482 0.389482 0.389482 0.394225 0.394225 0.394225 0.399381 0.399381 0.399381 0.405067 0.405067 0.405067 0.411413 0.411413 0.411413 0.418548 0.418548 0.418548 0.426565 0.426565 0.426565 0.435472 0.435472 0.435472 0.445133 0.445133 0.445133 0.45436 0.45436 0.45436 0.5 0.5 0.5 0.54564 0.54564 0.54564 0.554867 0.554867 0.554867 0.564528 0.564528 0.564528 0.573435 0.573435 0.573435 0.581452 0.581452 0.581452 0.588587 0.588587 0.588587 0.594933 0.594933 0.594933 0.600619 0.600619 0.600619 0.605775 0.605775 0.605775 0.610518 0.610518 0.610518 0.614948 0.614948 0.614948 0.619147 0.619147 0.619147 0.623181 0.623181 0.623181 0.627101 0.627101 0.627101 0.630952 0.630952 0.630952 0.634768 0.634768 0.634768 0.638576 0.638576 0.638576 0.6424 0.6424 0.6424 0.646258 0.646258 0.646258 0.650166 0.650166 0.650166 0.654136 0.654136 0.654136 0.65818 0.65818 0.65818 0.662306 0.662306 0.662306 0.666523 0.666523 0.666523 0.670836 0.670836 0.670836 0.690118 0.690118 0.690118 0.704708 0.704708 0.704708 0.720964 0.720964 0.720964 0.738885 0.738885 0.738885 0.758471 0.758471 0.758471 0.779723 0.779723 0.779723 0.80264 0.80264 0.80264 0.827222 0.827222 0.827222 0.85347 0.85347 0.85347 0.881383 0.881383 0.881383 0.910962 0.910962 0.910962 0.942205 0.942205 0.942205 1 1 1 1
  arc A210 (4.5056, 116.7321) -> (3.3515, 116.8466) centre (0.0435, 77.6158) ccw
  spline S9 degree 3 poles (0.3924, 116.9842) (0.4384, 116.8575) (0.4826, 116.73) (0.5247, 116.6019) (0.5475, 116.5326) (0.5696, 116.4632) (0.5912, 116.3935) (0.6115, 116.3276) (0.6314, 116.2614) (0.6506, 116.1951) (0.6687, 116.1326) (0.6863, 116.0699) (0.7033, 116.007) (0.7193, 115.9479) (0.7348, 115.8886) (0.7497, 115.8292) (0.7637, 115.7736) (0.7772, 115.7178) (0.7902, 115.662) (0.8024, 115.6099) (0.814, 115.5577) (0.8252, 115.5054) (0.8356, 115.4569) (0.8456, 115.4083) (0.8551, 115.3596) (0.8639, 115.3148) (0.8723, 115.2699) (0.8802, 115.2248) (0.8875, 115.1837) (0.8945, 115.1424) (0.901, 115.1011) (0.907, 115.0637) (0.9126, 115.0262) (0.9179, 114.9886) (0.9227, 114.9549) (0.9271, 114.9211) (0.9313, 114.8873) (0.9367, 114.8427) (0.9415, 114.7979) (0.9459, 114.7531) (0.9469, 114.7431) (0.9479, 114.7331) (0.949, 114.7231) (0.9501, 114.7133) (0.9512, 114.7036) (0.9525, 114.6938) (0.9537, 114.6842) (0.955, 114.6747) (0.9563, 114.6652) (0.9577, 114.6558) (0.9591, 114.6465) (0.9607, 114.6372) (0.9622, 114.628) (0.9638, 114.6189) (0.9654, 114.6098) (0.9671, 114.6008) (0.9689, 114.5919) (0.9707, 114.583) (0.9725, 114.5742) (0.9745, 114.5654) (0.9765, 114.5566) (0.9785, 114.5479) (0.9807, 114.5392) (0.9829, 114.5306) (0.9851, 114.522) (0.9875, 114.5134) (0.9899, 114.5049) (0.9924, 114.4963) (0.995, 114.4878) (0.9977, 114.4793) (1.0005, 114.4708) (1.0034, 114.4623) (1.0064, 114.4538) (1.0095, 114.4452) (1.0127, 114.4366) (1.0161, 114.4281) (1.0196, 114.4194) (1.0233, 114.4107) (1.0272, 114.4022) (1.0312, 114.3932) (1.0354, 114.3844) (1.0399, 114.3756) (1.0445, 114.3664) (1.0494, 114.3573) (1.0546, 114.3484) (1.0601, 114.3388) (1.0659, 114.3293) (1.072, 114.3201) (1.0787, 114.31) (1.0856, 114.3002) (1.0929, 114.2907) (1.101, 114.2801) (1.1095, 114.2699) (1.1184, 114.2601) (1.1283, 114.2491) (1.1388, 114.2385) (1.1497, 114.2285) (1.162, 114.2173) (1.1749, 114.2067) (1.1884, 114.1969) (1.2035, 114.1859) (1.2194, 114.1759) (1.2358, 114.1669) (1.254, 114.1569) (1.273, 114.1483) (1.2926, 114.1411) (1.3137, 114.1332) (1.3355, 114.127) (1.3577, 114.1229) (1.3788, 114.1189) (1.4003, 114.1167) (1.4218, 114.115) (1.5281, 114.1062) (1.6346, 114.1065) (1.741, 114.1015) (1.8474, 114.0966) (1.9535, 114.0864) (2.0601, 114.0853) (2.0817, 114.085) (2.1032, 114.0852) (2.1247, 114.0872) (2.1471, 114.0893) (2.1694, 114.0934) (2.1912, 114.0993) (2.2113, 114.1047) (2.231, 114.1115) (2.2501, 114.1197) (2.2673, 114.1271) (2.284, 114.1357) (2.3001, 114.1452) (2.3144, 114.1537) (2.3283, 114.163) (2.3416, 114.1731) (2.3534, 114.182) (2.3647, 114.1915) (2.3757, 114.2016) (2.3854, 114.2105) (2.3948, 114.2199) (2.4038, 114.2297) (2.412, 114.2385) (2.4199, 114.2476) (2.4274, 114.257) (2.4343, 114.2657) (2.441, 114.2745) (2.4474, 114.2836) (2.4533, 114.292) (2.4591, 114.3006) (2.4646, 114.3093) (2.4698, 114.3176) (2.4748, 114.3261) (2.4797, 114.3346) (2.4843, 114.3428) (2.4888, 114.3511) (2.4931, 114.3594) (2.4973, 114.3676) (2.5013, 114.3758) (2.5052, 114.3841) (2.509, 114.3922) (2.5126, 114.4004) (2.5162, 114.4087) (2.5197, 114.4169) (2.523, 114.4251) (2.5263, 114.4334) (2.5295, 114.4417) (2.5327, 114.45) (2.5357, 114.4583) (2.5387, 114.4667) (2.5416, 114.4752) (2.5445, 114.4836) (2.5473, 114.4922) (2.55, 114.5008) (2.5527, 114.5094) (2.5553, 114.5181) (2.5579, 114.5268) (2.5604, 114.5356) (2.5629, 114.5445) (2.5654, 114.5535) (2.5677, 114.5624) (2.5701, 114.5716) (2.5724, 114.5807) (2.5746, 114.5899) (2.5769, 114.5992) (2.579, 114.6086) (2.5811, 114.618) (2.5833, 114.6276) (2.5853, 114.6372) (2.5873, 114.6469) (2.5893, 114.6567) (2.5912, 114.6666) (2.5931, 114.6765) (2.6017, 114.7207) (2.6107, 114.7648) (2.6202, 114.8087) (2.6275, 114.842) (2.6351, 114.8752) (2.6429, 114.9083) (2.6517, 114.9452) (2.6608, 114.9821) (2.6702, 115.0188) (2.6805, 115.0593) (2.6913, 115.0997) (2.7024, 115.1401) (2.7145, 115.1841) (2.727, 115.2281) (2.7399, 115.2719) (2.7539, 115.3195) (2.7683, 115.367) (2.7832, 115.4143) (2.7992, 115.4653) (2.8157, 115.5162) (2.8326, 115.5669) (2.8507, 115.6214) (2.8693, 115.6756) (2.8884, 115.7297) (2.9088, 115.7875) (2.9297, 115.845) (2.9512, 115.9024) (2.9739, 115.9634) (2.9973, 116.0242) (3.0211, 116.0849) (3.0464, 116.1491) (3.0723, 116.2131) (3.0987, 116.2768) (3.1266, 116.3442) (3.1551, 116.4113) (3.1842, 116.4782) (3.2381, 116.6018) (3.2939, 116.7246) (3.3515, 116.8466) knots 0 0 0 0 0.057795 0.057795 0.057795 0.089038 0.089038 0.089038 0.118617 0.118617 0.118617 0.14653 0.14653 0.14653 0.172778 0.172778 0.172778 0.19736 0.19736 0.19736 0.220277 0.220277 0.220277 0.241529 0.241529 0.241529 0.261115 0.261115 0.261115 0.279036 0.279036 0.279036 0.295292 0.295292 0.295292 0.309882 0.309882 0.309882 0.329164 0.329164 0.329164 0.333477 0.333477 0.333477 0.337694 0.337694 0.337694 0.34182 0.34182 0.34182 0.345864 0.345864 0.345864 0.349834 0.349834 0.349834 0.353742 0.353742 0.353742 0.3576 0.3576 0.3576 0.361424 0.361424 0.361424 0.365232 0.365232 0.365232 0.369048 0.369048 0.369048 0.372899 0.372899 0.372899 0.376819 0.376819 0.376819 0.380853 0.380853 0.380853 0.385052 0.385052 0.385052 0.389482 0.389482 0.389482 0.394225 0.394225 0.394225 0.399381 0.399381 0.399381 0.405067 0.405067 0.405067 0.411413 0.411413 0.411413 0.418548 0.418548 0.418548 0.426565 0.426565 0.426565 0.435472 0.435472 0.435472 0.445133 0.445133 0.445133 0.45436 0.45436 0.45436 0.5 0.5 0.5 0.54564 0.54564 0.54564 0.554867 0.554867 0.554867 0.564528 0.564528 0.564528 0.573435 0.573435 0.573435 0.581452 0.581452 0.581452 0.588587 0.588587 0.588587 0.594933 0.594933 0.594933 0.600619 0.600619 0.600619 0.605775 0.605775 0.605775 0.610518 0.610518 0.610518 0.614948 0.614948 0.614948 0.619147 0.619147 0.619147 0.623181 0.623181 0.623181 0.627101 0.627101 0.627101 0.630952 0.630952 0.630952 0.634768 0.634768 0.634768 0.638576 0.638576 0.638576 0.6424 0.6424 0.6424 0.646258 0.646258 0.646258 0.650166 0.650166 0.650166 0.654136 0.654136 0.654136 0.65818 0.65818 0.65818 0.662306 0.662306 0.662306 0.666523 0.666523 0.666523 0.670836 0.670836 0.670836 0.690118 0.690118 0.690118 0.704708 0.704708 0.704708 0.720964 0.720964 0.720964 0.738885 0.738885 0.738885 0.758471 0.758471 0.758471 0.779723 0.779723 0.779723 0.80264 0.80264 0.80264 0.827222 0.827222 0.827222 0.85347 0.85347 0.85347 0.881383 0.881383 0.881383 0.910962 0.910962 0.910962 0.942205 0.942205 0.942205 1 1 1 1
  arc A211 (0.3924, 116.9842) -> (-0.7674, 116.9774) centre (0.0435, 77.6158) ccw
  spline S10 degree 3 poles (-3.7246, 116.805) (-3.6656, 116.6838) (-3.6084, 116.5616) (-3.5531, 116.4386) (-3.5232, 116.3721) (-3.4939, 116.3053) (-3.4652, 116.2383) (-3.4381, 116.1749) (-3.4114, 116.1112) (-3.3854, 116.0473) (-3.3608, 115.9869) (-3.3368, 115.9264) (-3.3133, 115.8656) (-3.2912, 115.8085) (-3.2696, 115.7512) (-3.2485, 115.6937) (-3.2288, 115.6398) (-3.2095, 115.5858) (-3.1908, 115.5316) (-3.1733, 115.4811) (-3.1562, 115.4304) (-3.1396, 115.3795) (-3.1242, 115.3324) (-3.1092, 115.2851) (-3.0947, 115.2377) (-3.0812, 115.194) (-3.0682, 115.1502) (-3.0556, 115.1063) (-3.044, 115.0661) (-3.0328, 115.0258) (-3.022, 114.9854) (-3.0121, 114.9488) (-3.0026, 114.9121) (-2.9934, 114.8753) (-2.9852, 114.8422) (-2.9772, 114.8091) (-2.9695, 114.7759) (-2.9595, 114.7321) (-2.95, 114.6881) (-2.9409, 114.644) (-2.9389, 114.6342) (-2.9369, 114.6243) (-2.9347, 114.6145) (-2.9327, 114.6049) (-2.9305, 114.5953) (-2.9282, 114.5857) (-2.926, 114.5763) (-2.9237, 114.567) (-2.9214, 114.5576) (-2.919, 114.5485) (-2.9166, 114.5394) (-2.9141, 114.5303) (-2.9117, 114.5213) (-2.9092, 114.5124) (-2.9065, 114.5035) (-2.9039, 114.4948) (-2.9013, 114.4861) (-2.8985, 114.4774) (-2.8957, 114.4688) (-2.8929, 114.4603) (-2.89, 114.4517) (-2.887, 114.4433) (-2.884, 114.4349) (-2.8809, 114.4266) (-2.8778, 114.4182) (-2.8746, 114.41) (-2.8712, 114.4017) (-2.8679, 114.3935) (-2.8644, 114.3853) (-2.8608, 114.3771) (-2.8572, 114.3689) (-2.8534, 114.3607) (-2.8495, 114.3526) (-2.8455, 114.3444) (-2.8414, 114.3362) (-2.8371, 114.3281) (-2.8327, 114.3198) (-2.8282, 114.3116) (-2.8234, 114.3035) (-2.8185, 114.295) (-2.8134, 114.2866) (-2.8081, 114.2784) (-2.8024, 114.2697) (-2.7966, 114.2612) (-2.7905, 114.2528) (-2.784, 114.2439) (-2.7773, 114.2351) (-2.7703, 114.2265) (-2.7626, 114.2172) (-2.7547, 114.2082) (-2.7464, 114.1994) (-2.7373, 114.1898) (-2.7278, 114.1805) (-2.7179, 114.1717) (-2.7068, 114.1618) (-2.6954, 114.1524) (-2.6834, 114.1436) (-2.67, 114.1337) (-2.6561, 114.1246) (-2.6417, 114.1162) (-2.6255, 114.1069) (-2.6087, 114.0985) (-2.5914, 114.0913) (-2.5722, 114.0833) (-2.5524, 114.0767) (-2.5322, 114.0716) (-2.5103, 114.066) (-2.488, 114.0621) (-2.4655, 114.0602) (-2.4441, 114.0585) (-2.4225, 114.0586) (-2.401, 114.0591) (-2.2944, 114.0615) (-2.1884, 114.0729) (-2.0821, 114.0791) (-1.9758, 114.0853) (-1.8692, 114.0863) (-1.763, 114.0963) (-1.7416, 114.0983) (-1.7201, 114.1007) (-1.699, 114.1049) (-1.6769, 114.1094) (-1.6552, 114.1158) (-1.6341, 114.1239) (-1.6147, 114.1314) (-1.5958, 114.1402) (-1.5777, 114.1504) (-1.5614, 114.1596) (-1.5456, 114.1698) (-1.5306, 114.181) (-1.5173, 114.1909) (-1.5045, 114.2017) (-1.4923, 114.213) (-1.4815, 114.2232) (-1.4712, 114.2338) (-1.4614, 114.2449) (-1.4526, 114.2549) (-1.4442, 114.2652) (-1.4363, 114.2758) (-1.4291, 114.2855) (-1.4222, 114.2954) (-1.4157, 114.3055) (-1.4097, 114.3148) (-1.404, 114.3243) (-1.3986, 114.334) (-1.3936, 114.343) (-1.3888, 114.3521) (-1.3842, 114.3614) (-1.3799, 114.3702) (-1.3758, 114.3791) (-1.3718, 114.3881) (-1.3681, 114.3967) (-1.3645, 114.4054) (-1.3611, 114.4142) (-1.3578, 114.4227) (-1.3547, 114.4313) (-1.3517, 114.44) (-1.3487, 114.4485) (-1.3459, 114.457) (-1.3433, 114.4656) (-1.3407, 114.4741) (-1.3382, 114.4826) (-1.3358, 114.4912) (-1.3334, 114.4998) (-1.3312, 114.5084) (-1.3291, 114.517) (-1.3269, 114.5257) (-1.3249, 114.5344) (-1.323, 114.5431) (-1.3211, 114.5519) (-1.3192, 114.5607) (-1.3175, 114.5695) (-1.3158, 114.5785) (-1.3141, 114.5875) (-1.3126, 114.5964) (-1.311, 114.6056) (-1.3095, 114.6147) (-1.3081, 114.6239) (-1.3067, 114.6332) (-1.3053, 114.6425) (-1.3041, 114.6519) (-1.3028, 114.6614) (-1.3017, 114.671) (-1.3005, 114.6806) (-1.2994, 114.6903) (-1.2984, 114.7001) (-1.2974, 114.7099) (-1.2965, 114.7199) (-1.2956, 114.73) (-1.2947, 114.74) (-1.2908, 114.7848) (-1.2865, 114.8296) (-1.2816, 114.8743) (-1.2779, 114.9082) (-1.2738, 114.942) (-1.2695, 114.9758) (-1.2646, 115.0134) (-1.2594, 115.051) (-1.2539, 115.0885) (-1.2478, 115.1299) (-1.2414, 115.1712) (-1.2346, 115.2124) (-1.2271, 115.2575) (-1.2192, 115.3026) (-1.211, 115.3475) (-1.2021, 115.3963) (-1.1927, 115.445) (-1.1828, 115.4936) (-1.1723, 115.546) (-1.1612, 115.5983) (-1.1497, 115.6506) (-1.1373, 115.7066) (-1.1245, 115.7625) (-1.1111, 115.8183) (-1.0969, 115.8779) (-1.0821, 115.9373) (-1.0668, 115.9966) (-1.0505, 116.0597) (-1.0337, 116.1226) (-1.0163, 116.1854) (-0.9979, 116.2519) (-0.9788, 116.3182) (-0.9592, 116.3844) (-0.9385, 116.4543) (-0.9172, 116.524) (-0.8952, 116.5936) (-0.8546, 116.7222) (-0.8119, 116.8501) (-0.7674, 116.9774) knots 0 0 0 0 0.057795 0.057795 0.057795 0.089038 0.089038 0.089038 0.118617 0.118617 0.118617 0.14653 0.14653 0.14653 0.172778 0.172778 0.172778 0.19736 0.19736 0.19736 0.220277 0.220277 0.220277 0.241529 0.241529 0.241529 0.261115 0.261115 0.261115 0.279036 0.279036 0.279036 0.295292 0.295292 0.295292 0.309882 0.309882 0.309882 0.329164 0.329164 0.329164 0.333477 0.333477 0.333477 0.337694 0.337694 0.337694 0.34182 0.34182 0.34182 0.345864 0.345864 0.345864 0.349834 0.349834 0.349834 0.353742 0.353742 0.353742 0.3576 0.3576 0.3576 0.361424 0.361424 0.361424 0.365232 0.365232 0.365232 0.369048 0.369048 0.369048 0.372899 0.372899 0.372899 0.376819 0.376819 0.376819 0.380853 0.380853 0.380853 0.385052 0.385052 0.385052 0.389482 0.389482 0.389482 0.394225 0.394225 0.394225 0.399381 0.399381 0.399381 0.405067 0.405067 0.405067 0.411413 0.411413 0.411413 0.418548 0.418548 0.418548 0.426565 0.426565 0.426565 0.435472 0.435472 0.435472 0.445133 0.445133 0.445133 0.45436 0.45436 0.45436 0.5 0.5 0.5 0.54564 0.54564 0.54564 0.554867 0.554867 0.554867 0.564528 0.564528 0.564528 0.573435 0.573435 0.573435 0.581452 0.581452 0.581452 0.588587 0.588587 0.588587 0.594933 0.594933 0.594933 0.600619 0.600619 0.600619 0.605775 0.605775 0.605775 0.610518 0.610518 0.610518 0.614948 0.614948 0.614948 0.619147 0.619147 0.619147 0.623181 0.623181 0.623181 0.627101 0.627101 0.627101 0.630952 0.630952 0.630952 0.634768 0.634768 0.634768 0.638576 0.638576 0.638576 0.6424 0.6424 0.6424 0.646258 0.646258 0.646258 0.650166 0.650166 0.650166 0.654136 0.654136 0.654136 0.65818 0.65818 0.65818 0.662306 0.662306 0.662306 0.666523 0.666523 0.666523 0.670836 0.670836 0.670836 0.690118 0.690118 0.690118 0.704708 0.704708 0.704708 0.720964 0.720964 0.720964 0.738885 0.738885 0.738885 0.758471 0.758471 0.758471 0.779723 0.779723 0.779723 0.80264 0.80264 0.80264 0.827222 0.827222 0.827222 0.85347 0.85347 0.85347 0.881383 0.881383 0.881383 0.910962 0.910962 0.910962 0.942205 0.942205 0.942205 1 1 1 1
  arc A212 (-3.7246, 116.805) -> (-4.8774, 116.677) centre (0.0435, 77.6158) ccw